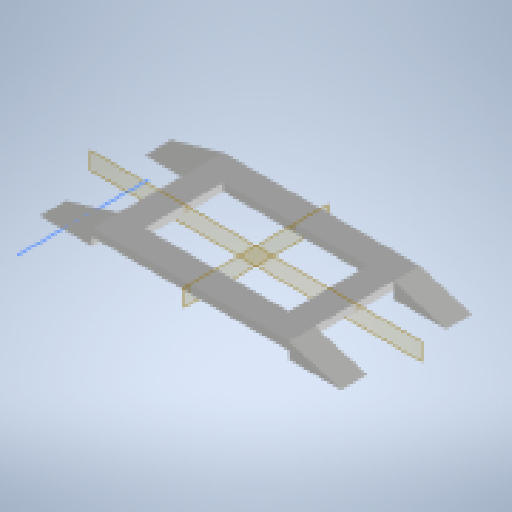
# Autodesk Inventor part: Base_plartform
Saved by Autodesk Inventor 2023 (Build 270158000, 158)
## iProperties
Created: 2023-11-19
Part Number: Base_plartform
Material: Stainless Steel
Document SubType Name: Modeling
Designer: Beatrice
Density: 8 g/cm^3
Appearance: Silver
Author: Beatrice
Autodesk Inventor part; units mm, degrees
ref_plane "YZ Plane" through (0, 0, 0) normal (1, 0, 0) x (0, 1, 0)
ref_plane "XZ Plane" through (0, 0, 0) normal (0, 1, 0) x (-1, 0, 0)
sketch "Sketch1" plane through (0, 0, 0) normal (0, 0, 1) x (1, 0, 0)
  line L0 (137.5, -75) -> (-137.5, -75)
  line L1 (-137.5, -75) -> (-137.5, 75)
  line L2 (-137.5, 75) -> (137.5, 75)
  line L3 (137.5, 75) -> (137.5, -75)
  line L4 (137.5, -75) -> (-137.5, 75) construction
  line L5 (-137.5, -75) -> (137.5, 75) construction
  line L6 (187.5, 125) -> (-187.5, 125)
  line L7 (-187.5, 125) -> (-187.5, -125)
  line L8 (-187.5, -125) -> (187.5, -125)
  line L9 (187.5, -125) -> (187.5, 125)
  line L10 (-187.5, 125) -> (-287.5, 125)
  line L11 (-287.5, 125) -> (-287.5, 75)
  line L12 (-287.5, 75) -> (-187.5, 75)
  line L13 (-187.5, 75) -> (-187.5, 125)
  line L14 (-187.5, -75) -> (-287.5, -75)
  line L15 (-287.5, -75) -> (-287.5, -125)
  line L16 (-287.5, -125) -> (-187.5, -125)
  line L17 (-187.5, -125) -> (-187.5, -75)
  line L18 (0, 175) -> (0, -175) construction
  line L19 (-1719.5601, 0) -> (1799.9601, 0) construction
  line L20 (187.5, 125) -> (287.5, 125)
  line L21 (287.5, 125) -> (287.5, 75)
  line L22 (287.5, 75) -> (187.5, 75)
  line L23 (187.5, -75) -> (287.5, -75)
  line L24 (287.5, -75) -> (287.5, -125)
  line L25 (287.5, -125) -> (187.5, -125)
  line L26 (1719.5601, 0) -> (-1799.9601, 0) construction
  point P0 (0, 0)
  point P1 (237.5, -125)
  point P2 (0, -125)
  point P3 (-237.5, 125)
  point P4 (0, 125)
  point P5 (237.5, 125)
  point P6 (-237.5, -125)
  point P7 (-237.5, -75)
  point P8 (0, -75)
  point P9 (-237.5, 75)
  point P10 (0, 75)
  point P11 (-287.5, 100)
  point P12 (-287.5, -100)
  point P13 (287.5, 100)
  point P14 (287.5, -100)
  point P15 (187.5, 75)
  dimension "d0" = 50
  dimension "d1" = 150
  dimension "d2" = 275
  dimension "d3" = 100
  constraints: 50 end point, 16 midpoint, 9 symmetric about line, 8 parallel, 6 horizontal alignment, 4 perpendicular, 3 horizontal, 3 point on line, 2 vertical alignment, 3 other
  measures "d0" distance between parallel lines of L2 L6
  measures "d1" distance of L0.end L1.end
  measures "d2" distance of L0.start L0.end
  measures "d3" distance of L6.end L10.end
extrude "Extrusion1" add sketch "Sketch1" along normal blind 30
ref_plane "Work Plane1" through (-287.5, 0, 0) normal (0, -1, 0) x (1, 0, 0)
sketch "Sketch2" plane through (-287.5, 0, 0) normal (0, -1, 0) x (1, 0, 0)
  line L0 (475, 30) -> (475, 0) construction
  line L1 (475, 0) -> (425, 0) construction
  line L2 (425, 0) -> (425, 30) construction
  line L3 (425, 30) -> (475, 30) construction
  line L4 (100, 0) -> (100, 30) construction
  line L5 (100, 30) -> (150, 30) construction
  line L6 (150, 30) -> (150, 0) construction
  line L7 (150, 0) -> (100, 0) construction
  line L8 (475, 30) -> (475, 0) construction
  line L9 (475, 0) -> (425, 0) construction
  line L10 (425, 0) -> (425, 30) construction
  line L11 (100, 0) -> (100, 30) construction
  line L12 (150, 30) -> (150, 0) construction
  line L13 (150, 0) -> (100, 0) construction
  line L14 (0, 0) -> (100, 0) construction
  line L15 (100, 0) -> (100, 30) construction
  line L16 (0, 30) -> (100, 30) construction
  line L17 (0, 0) -> (0, 30) construction
  line L18 (150, 0) -> (425, 0) construction
  line L19 (425, 0) -> (425, 30) construction
  line L20 (150, 30) -> (425, 30) construction
  line L21 (150, 0) -> (150, 30) construction
  line L22 (475, 0) -> (575, 0) construction
  line L23 (575, 0) -> (575, 30) construction
  line L24 (475, 30) -> (575, 30) construction
  line L25 (475, 0) -> (475, 30) construction
  line L26 (0, 0) -> (0, 30) projected
  line L27 (0, 0) -> (100, 30)
  line L28 (475, 30) -> (575, 0)
  line L29 (425, 30) -> (475, 30) projected
  line L30 (100, 30) -> (150, 30) projected
  line L31 (0, 0) -> (100, 0)
  line L32 (100, 30) -> (100, 0)
  line L33 (475, 30) -> (475, 0)
  line L34 (575, 0) -> (0, 0) projected
  line L35 (575, 0) -> (475, 0)
  line L36 (0, 30) -> (100, 30)
  line L37 (100, 30) -> (100, 0)
  line L38 (100, 0) -> (0, 0)
  line L39 (0, 0) -> (0, 30)
  line L40 (475, 30) -> (575, 30)
  line L41 (575, 30) -> (575, 0)
  line L42 (575, 0) -> (475, 0)
  line L43 (475, 0) -> (475, 30)
  point P0 (287.5, 0)
  constraints: 28 end point, 5 parallel, 3 horizontal, 2 collinear, 2 perpendicular, 1 other
extrude "Extrusion2" cut sketch "Sketch2" along normal through all both and the other way through all contours L26 L36 L27 | L40 L41 L28
sketch "Sketch3" plane through (-287.5, -125, 0) normal (0, -1, 0) x (1, 0, 0)
  line L0 (475, 0) -> (475, 30) projected
  line L1 (100, 0) -> (475, 0)
  line L2 (475, 0) -> (475, 15)
  line L3 (475, 15) -> (100, 15)
  line L4 (100, 15) -> (100, 0)
  line L5 (0, 0) -> (575, 0) projected
  point P0 (287.5, 0)
  point P1 (287.5, 0)
  constraints: 8 end point, 3 midpoint, 2 parallel, 1 horizontal, 1 perpendicular
extrude "Extrusion3" cut sketch "Sketch3" against normal through all
ref_plane "Work Plane2" through (-187.5, 0, 30) normal (0, -1, 0) x (1, 0, 0)
ref_plane "Work Plane3" through (0, -75, 30) normal (1, 0, 0) x (0, 0, -1)
body "Solid1"
